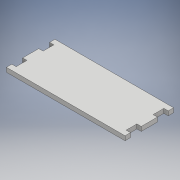
# Autodesk Inventor part: FUENTE 1
Saved by Autodesk Inventor 2018 (Build 220112000, 112)
## iProperties
Created: 2018-03-06
Part Number: FUENTE 1
Material: Generic
Document SubType Name: Modeling
Designer: isai
Density: 1 g/cm^3
Appearance: Default
Author: isai
Autodesk Inventor part; units mm, degrees
ref_plane "YZ Plane" through (0, 0, 0) normal (1, 0, 0) x (0, 1, 0)
ref_plane "XZ Plane" through (0, 0, 0) normal (0, 1, 0) x (-1, 0, 0)
ref_plane "XY Plane" through (0, 0, 0) normal (0, 0, 1) x (1, 0, 0)
sketch "Sketch1" plane through (0, 0, 0) normal (0, 0, 1) x (1, 0, 0)
  line L0 (55, -22.5) -> (-55, -22.5)
  line L1 (-55, -22.5) -> (-55, 22.5)
  line L2 (-55, 22.5) -> (55, 22.5)
  line L3 (55, 22.5) -> (55, -22.5)
  line L4 (55, -22.5) -> (-55, 22.5) construction
  line L5 (-55, -22.5) -> (55, 22.5) construction
  point P0 (0, 0)
  dimension "d0" = 110
  dimension "d1" = 45
  constraints: 12 end point, 2 midpoint, 2 parallel, 1 horizontal, 1 perpendicular
  measures "d0" distance of L1.end L2.end
  measures "d1" distance of L2.end L0.start
extrude "Extrusion1" add sketch "Sketch1" along normal blind 4
sketch "Sketch2" plane through (0, 0, 4) normal (0, 0, 1) x (1, 0, 0)
  line L0 (-55, 22.5) -> (-55, -22.5) projected
  line L1 (-55, 17.5) -> (-51, 17.5)
  line L2 (-51, 17.5) -> (-51, 7.5)
  line L3 (-51, 7.5) -> (-55, 7.5)
  line L4 (-55, 7.5) -> (-55, 17.5)
  line L5 (-55, -7.5) -> (-51, -7.5)
  line L6 (-51, -7.5) -> (-51, -17.5)
  line L7 (-51, -17.5) -> (-55, -17.5)
  line L8 (-55, -17.5) -> (-55, -7.5)
  line L9 (55, 22.5) -> (-55, 22.5) projected
  line L10 (-55, -22.5) -> (55, -22.5) projected
  point P0 (0, 0)
  dimension "d4" = 4
  dimension "d5" = 10
  dimension "d6" = 4
  dimension "d7" = 10
  dimension "d8" = 5
  dimension "d9" = 5
  constraints: 16 end point, 4 parallel, 2 horizontal, 2 perpendicular, 2 point on line
  measures "d4" distance of L2.end L3.end
  measures "d5" distance of L1.end L2.end
  measures "d6" distance of L6.end L7.end
  measures "d7" distance of L5.end L6.end
  measures "d8" distance between parallel lines of L1 L9
  measures "d9" distance between parallel lines of L7 L10
extrude "Extrusion2" cut sketch "Sketch2" against normal blind 4
ref_plane "Work Plane2" through (0, -7.5, 0) normal (-1, 0, 0) x (0, 0, 1)
mirror "Mirror1" about plane through (0, -7.5, 0) normal (-1, 0, 0) of "Extrusion2"
body "Solid1"
